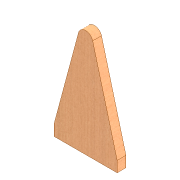
# Autodesk Inventor part: CPO-1-support
Saved by Autodesk Inventor 2020 (Build 240168000, 168)
## iProperties
Created: 2021-06-30
Part Number: CPO-1-support
Material: Generic
Document SubType Name: Modeling
Designer: Aidan Lee
Density: 1 g/cm^3
Appearance: Cherry - Natural Low Gloss
Author: Aidan Lee
Autodesk Inventor part; units mm, degrees
ref_plane "YZ Plane" through (0, 0, 0) normal (1, 0, 0) x (0, 1, 0)
ref_plane "XZ Plane" through (0, 0, 0) normal (0, 1, 0) x (-1, 0, 0)
ref_plane "XY Plane" through (0, 0, 0) normal (0, 0, 1) x (1, 0, 0)
sketch "Sketch1" plane through (0, 0, 0) normal (0, 0, 1) x (1, 0, 0)
  line L0 (0, 0) -> (219, 0) construction
  line L1 (219, 0) -> (219, 18) construction
  line L2 (219, 18) -> (0, 18) construction
  line L3 (0, 18) -> (0, 0) construction
  line L4 (44.9362, 18) -> (174.0638, 18)
  line L5 (174.0638, 18) -> (174.0638, 40)
  line L6 (174.0638, 40) -> (44.9362, 40) construction
  line L7 (44.9362, 40) -> (44.9362, 18)
  line L8 (91.5484, 238) -> (127.4516, 238) construction
  arc A0 (123.9889, 226.8823) -> (95.0111, 226.8823) centre (109.5, 223) ccw
  line L9 (109.5, 238) -> (109.5, 292.3651) construction
  line L10 (44.9362, 40) -> (95.0111, 226.8823)
  line L11 (174.0638, 40) -> (123.9889, 226.8823)
  point P0 (109.5, 40)
  point P1 (109.5, 0)
  dimension "d2" = 18
  dimension "d3" = 219
  dimension "d4" = 40
  dimension "d5" = 220
  dimension "d6" = 15
  dimension "d7" = 75
  constraints: 24 end point, 4 parallel, 3 horizontal, 3 midpoint, 3 point on circle, 3 vertical alignment, 2 perpendicular, 1 centre point, 1 horizontal alignment, 1 point on line, 1 tangent, 1 vertical
  measures "d2" distance of L2.end L0.start
  measures "d3" distance of L0.start L0.end
  measures "d4" distance between parallel lines of L0 L6
  measures "d5" distance between parallel lines of L8 L2
  measures "d6" radius of A0
  measures "d7" angle of L10 L6
extrude "Extrusion1" add sketch "Sketch1" along normal blind 18
body "Solid1"
